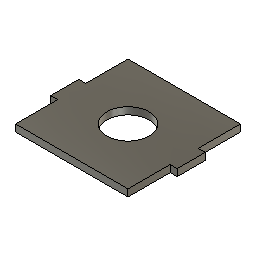
Activity3Solution v3 (Autodesk Fusion 360 design; units mm, degrees)
Autodesk Fusion 360 part; units mm, degrees
sketch "Sketch1" plane through (0, 0, 0) normal (0, 0, 1) x (1, 0, 0)
  line L0 (21.6826, 76.2435) -> (61.6826, 76.2435)
  line L1 (61.6826, 76.2435) -> (61.6826, 61.2435)
  line L2 (21.6826, 76.2435) -> (21.6826, 61.2435)
  line L3 (61.6826, 61.2435) -> (64.1826, 61.2435)
  line L4 (21.6826, 61.2435) -> (19.1826, 61.2435)
  line L5 (64.1826, 61.2435) -> (64.1826, 51.2435)
  line L6 (19.1826, 61.2435) -> (19.1826, 51.2435)
  line L7 (64.1826, 51.2435) -> (61.6826, 51.2435)
  line L8 (19.1826, 51.2435) -> (21.6826, 51.2435)
  line L9 (21.6826, 51.2435) -> (21.6826, 36.2435)
  line L10 (61.6826, 51.2435) -> (61.6826, 36.2435)
  line L11 (61.6826, 36.2435) -> (21.6826, 36.2435)
  circle A0 centre (41.6826, 56.2435) radius 7.5
  dimension "d1" = 40
  dimension "d2" = 15
  dimension "d3" = 15
  dimension "d4" = 2.5
  dimension "d5" = 2.5
  dimension "d6" = 10
  dimension "d7" = 10
  dimension "d8" = 2.5
  dimension "d9" = 2.5
  dimension "d10" = 15
  dimension "d11" = 15
  dimension "d12" = 15
  dimension "d13" = 20
  dimension "d14" = 22.5
  constraint horizontal L0
  constraint perpendicular L0 L1
  constraint perpendicular L0 L2
  constraint horizontal L3
  constraint horizontal L4
  constraint perpendicular L3 L5
  constraint perpendicular L4 L6
  constraint perpendicular L5 L7
  constraint perpendicular L6 L8
  constraint perpendicular L8 L9
  constraint perpendicular L7 L10
  measures "d1" distance of L0.start L0.end
  measures "d2" distance of L0.end L1.end
  measures "d3" distance of L0.start L2.end
  measures "d4" distance of L1.end L3.end
  measures "d5" distance of L2.end L4.end
  measures "d6" distance of L3.end L5.end
  measures "d7" distance of L4.end L6.end
  measures "d8" distance of L5.end L7.end
  measures "d9" distance of L6.end L8.end
  measures "d10" distance of L8.end L9.end
  measures "d11" distance of L7.end L10.end
  measures "d12" diameter of A0
  measures "d13" distance of L0 A0.centre
  measures "d14" distance of L5 A0.centre
extrude "Extrude1" add sketch "Sketch1" along normal blind 2.5
